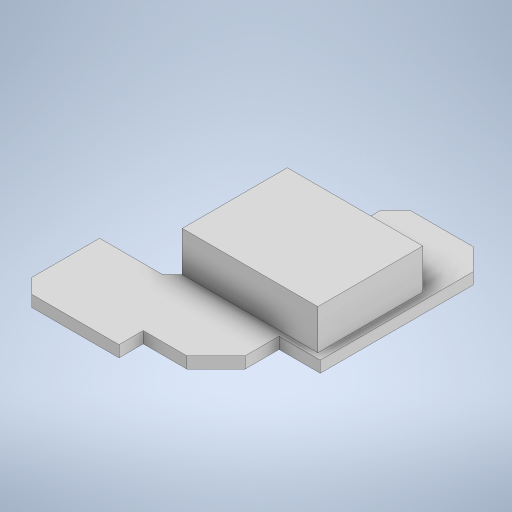
# Autodesk Inventor part: touch_pcb
Saved by Autodesk Inventor 2023 (Build 270158000, 158)
## iProperties
Created: 2023-03-12
Part Number: touch_pcb
Material: Generic
Document SubType Name: Modeling
Designer: nigel
Density: 1 g/cm^3
Appearance: Default
Author: nigel
Autodesk Inventor part; units mm, degrees
(part 1 of 2)
ref_plane "YZ Plane" through (0, 0, 0) normal (1, 0, 0) x (0, 1, 0)
ref_plane "XZ Plane" through (0, 0, 0) normal (0, 1, 0) x (-1, 0, 0)
sketch "Sketch1" plane through (0, 0, 0) normal (0, 1, 0) x (-1, 0, 0)
  arc A0 (8.4542, 10.3296) -> (8.3798, 10.2604) centre (8.417, 10.295) ccw
  arc A1 (10.1943, 12.5176) -> (10.1224, 12.5895) centre (10.1584, 12.5535) ccw
  arc A2 (8.7439, 11.2109) -> (8.8157, 11.1391) centre (8.7798, 11.175) ccw
  line L0 (10.1584, 12.5536) -> (8.7798, 11.175)
  arc A3 (8.7798, 11.1242) -> (8.7798, 11.2258) centre (8.7798, 11.175) ccw
  arc A4 (4.4414, 11.2258) -> (4.4414, 11.1242) centre (4.4414, 11.175) ccw
  line L1 (8.7798, 11.175) -> (4.4414, 11.175)
  arc A5 (4.4773, 11.1391) -> (4.4055, 11.2109) centre (4.4414, 11.175) ccw
  arc A6 (3.7865, 10.5919) -> (3.8583, 10.5201) centre (3.8224, 10.556) ccw
  line L2 (4.4414, 11.175) -> (3.8224, 10.556)
  arc A7 (3.8732, 10.556) -> (3.7716, 10.556) centre (3.8224, 10.556) ccw
  line L3 (3.8224, 10.556) -> (3.8224, 9.6448)
  arc A8 (10.1731, 10.4919) -> (10.1469, 10.5901) centre (10.16, 10.541) ccw
  arc A9 (9.053, 10.2987) -> (9.0792, 10.2005) centre (9.0661, 10.2496) ccw
  line L4 (10.16, 10.541) -> (9.0661, 10.2496)
  arc A10 (8.422, 10.215) -> (8.4964, 10.2842) centre (8.4592, 10.2496) ccw
  arc A11 (2.8503, 9.2057) -> (2.7785, 9.2775) centre (2.8144, 9.2416) ccw
  line L5 (8.4592, 10.2496) -> (8.417, 10.295)
  arc A12 (9.0661, 10.1988) -> (9.0661, 10.3004) centre (9.0661, 10.2496) ccw
  arc A13 (8.4592, 10.3004) -> (8.4592, 10.1988) centre (8.4592, 10.2496) ccw
  line L6 (9.0661, 10.2496) -> (8.4592, 10.2496)
  arc A14 (7.6178, 12.895) -> (7.5162, 12.895) centre (7.567, 12.895) ccw
  line L7 (7.567, 11.684) -> (7.567, 12.895)
  arc A15 (4.318, 11.7348) -> (4.318, 11.6332) centre (4.318, 11.684) ccw
  arc A16 (7.567, 11.6332) -> (7.567, 11.7348) centre (7.567, 11.684) ccw
  line L8 (4.318, 11.684) -> (7.567, 11.684)
  arc A17 (3.2781, 10.7159) -> (3.3499, 10.6441) centre (3.314, 10.68) ccw
  arc A18 (4.3539, 11.6481) -> (4.2821, 11.7199) centre (4.318, 11.684) ccw
  line L9 (3.314, 10.68) -> (4.318, 11.684)
  arc A19 (3.2632, 9.485) -> (3.3648, 9.485) centre (3.314, 9.485) ccw
  arc A20 (3.3648, 10.68) -> (3.2632, 10.68) centre (3.314, 10.68) ccw
  line L10 (3.314, 9.485) -> (3.314, 10.68)
  arc A21 (3.7716, 9.6448) -> (3.8732, 9.6448) centre (3.8224, 9.6448) ccw
  arc A22 (1.9961, 8.4951) -> (2.0679, 8.4233) centre (2.032, 8.4592) ccw
  line L11 (2.8144, 9.2416) -> (2.032, 8.4592)
  arc A23 (1.454, 1.1071) -> (1.5259, 1.1789) centre (1.4899, 1.143) ccw
  arc A24 (0.5852, 2.1196) -> (0.5134, 2.0477) centre (0.5493, 2.0837) ccw
  line L12 (1.49, 1.143) -> (0.5493, 2.0837)
  arc A25 (1.651, 1.0922) -> (1.651, 1.1938) centre (1.651, 1.143) ccw
  arc A26 (1.49, 1.1938) -> (1.49, 1.0922) centre (1.49, 1.143) ccw
  line L13 (1.651, 1.143) -> (1.49, 1.143)
  arc A27 (2.0679, 5.3321) -> (1.9961, 5.404) centre (2.032, 5.3681) ccw
  arc A28 (0.5134, 3.9213) -> (0.5852, 3.8494) centre (0.5493, 3.8854) ccw
  line L14 (2.032, 5.368) -> (0.5493, 3.8853)
  arc A29 (0.6001, 3.8853) -> (0.4985, 3.8853) centre (0.5493, 3.8853) ccw
  arc A30 (0.4985, 2.0837) -> (0.6001, 2.0837) centre (0.5493, 2.0837) ccw
  line L15 (0.5493, 3.8853) -> (0.5493, 2.0837)
  arc A31 (2.0828, 8.4592) -> (1.9812, 8.4592) centre (2.032, 8.4592) ccw
  arc A32 (1.9812, 5.368) -> (2.0828, 5.368) centre (2.032, 5.368) ccw
  line L16 (2.032, 8.4592) -> (2.032, 5.368)
  arc A33 (2.7636, 9.4427) -> (2.8652, 9.4437) centre (2.8144, 9.4432) ccw
  arc A34 (2.8648, 9.4855) -> (2.7632, 9.4845) centre (2.814, 9.485) ccw
  line L17 (2.8144, 9.4432) -> (2.814, 9.485)
  arc A35 (2.8652, 9.4432) -> (2.7636, 9.4432) centre (2.8144, 9.4432) ccw
  arc A36 (2.7636, 9.2416) -> (2.8652, 9.2416) centre (2.8144, 9.2416) ccw
  line L18 (2.8144, 9.4432) -> (2.8144, 9.2416)
  arc A37 (6.7529, 12.3511) -> (6.6811, 12.4229) centre (6.717, 12.387) ccw
  arc A38 (6.4025, 12.1443) -> (6.4743, 12.0725) centre (6.4384, 12.1084) ccw
  line L19 (6.717, 12.387) -> (6.4384, 12.1084)
  arc A39 (6.6662, 12.387) -> (6.7678, 12.387) centre (6.717, 12.387) ccw
  arc A40 (6.7678, 12.895) -> (6.6662, 12.895) centre (6.717, 12.895) ccw
  line L20 (6.717, 12.387) -> (6.717, 12.895)
  arc A41 (2.865, 10.9359) -> (2.7634, 10.9359) centre (2.8142, 10.9359) ccw
  arc A42 (2.7632, 9.485) -> (2.8648, 9.485) centre (2.814, 9.485) ccw
  line L21 (2.8142, 10.9359) -> (2.814, 9.485)
  arc A43 (4.019, 12.0725) -> (3.947, 12.1443) centre (3.983, 12.1084) ccw
  arc A44 (2.7782, 10.9717) -> (2.8502, 10.9) centre (2.8142, 10.9359) ccw
  line L22 (3.983, 12.1084) -> (2.8142, 10.9359)
  arc A45 (1.6151, 3.2109) -> (1.6869, 3.1391) centre (1.651, 3.175) ccw
  arc A46 (3.983, 12.1592) -> (3.983, 12.0576) centre (3.983, 12.1084) ccw
  line L23 (6.4384, 12.1084) -> (3.983, 12.1084)
  arc A47 (7.5162, 11.684) -> (7.6178, 11.684) centre (7.567, 11.684) ccw
  arc A48 (6.4384, 12.0576) -> (6.4384, 12.1592) centre (6.4384, 12.1084) ccw
  arc A49 (2.7696, 4.2218) -> (2.6978, 4.2936) centre (2.7337, 4.2577) ccw
  line L24 (2.7337, 4.2577) -> (1.651, 3.175)
  arc A50 (2.7845, 7.1723) -> (2.6829, 7.1723) centre (2.7337, 7.1723) ccw
  arc A51 (2.6829, 4.2577) -> (2.7845, 4.2577) centre (2.7337, 4.2577) ccw
  line L25 (2.7337, 7.1723) -> (2.7337, 4.2577)
  arc A52 (4.3499, 8.7167) -> (4.2781, 8.7885) centre (4.314, 8.7526) ccw
  arc A53 (2.6978, 7.2082) -> (2.7696, 7.1364) centre (2.7337, 7.1723) ccw
  line L26 (4.314, 8.7526) -> (2.7337, 7.1723)
  arc A54 (4.3648, 9.485) -> (4.2632, 9.485) centre (4.314, 9.485) ccw
  arc A55 (4.2632, 8.7526) -> (4.3648, 8.7526) centre (4.314, 8.7526) ccw
  line L27 (4.314, 9.485) -> (4.314, 8.7526)
  arc A56 (4.314, 10.3458) -> (4.314, 10.2442) centre (4.314, 10.295) ccw
  arc A57 (6.717, 10.2442) -> (6.717, 10.3458) centre (6.717, 10.295) ccw
  line L28 (4.314, 10.295) -> (6.717, 10.295)
  arc A58 (4.2632, 9.485) -> (4.3648, 9.485) centre (4.314, 9.485) ccw
  arc A59 (4.3648, 10.295) -> (4.2632, 10.295) centre (4.314, 10.295) ccw
  line L29 (4.314, 9.485) -> (4.314, 10.295)
  arc A60 (4.9689, 2.3571) -> (4.8971, 2.4289) centre (4.933, 2.393) ccw
  arc A61 (3.6471, 1.1789) -> (3.7189, 1.1071) centre (3.683, 1.143) ccw
  line L30 (4.933, 2.393) -> (3.683, 1.143)
  arc A62 (4.9838, 7.072) -> (4.8822, 7.072) centre (4.933, 7.072) ccw
  arc A63 (4.8822, 2.393) -> (4.9838, 2.393) centre (4.933, 2.393) ccw
  line L31 (4.933, 7.072) -> (4.933, 2.393)
  arc A64 (5.3499, 7.4171) -> (5.2781, 7.4889) centre (5.314, 7.453) ccw
  arc A65 (4.8971, 7.1079) -> (4.9689, 7.0361) centre (4.933, 7.072) ccw
  line L32 (5.314, 7.453) -> (4.933, 7.072)
  arc A66 (5.3648, 9.485) -> (5.2632, 9.485) centre (5.314, 9.485) ccw
  arc A67 (5.2632, 7.453) -> (5.3648, 7.453) centre (5.314, 7.453) ccw
  line L33 (5.314, 9.485) -> (5.314, 7.453)
  arc A68 (3.7338, 6.731) -> (3.6322, 6.731) centre (3.683, 6.731) ccw
  arc A69 (3.6322, 3.175) -> (3.7338, 3.175) centre (3.683, 3.175) ccw
  line L34 (3.683, 6.731) -> (3.683, 3.175)
  arc A70 (4.8663, 7.8425) -> (4.7945, 7.9143) centre (4.8304, 7.8784) ccw
  arc A71 (3.6471, 6.7669) -> (3.7189, 6.6951) centre (3.683, 6.731) ccw
  line L35 (4.8304, 7.8784) -> (3.683, 6.731)
  arc A72 (4.8812, 9.4686) -> (4.7796, 9.4686) centre (4.8304, 9.4686) ccw
  arc A73 (4.7796, 7.8784) -> (4.8812, 7.8784) centre (4.8304, 7.8784) ccw
  line L36 (4.8304, 9.4686) -> (4.8304, 7.8784)
  arc A74 (4.8499, 9.5209) -> (4.7781, 9.4491) centre (4.814, 9.485) ccw
  arc A75 (4.7945, 9.4327) -> (4.8663, 9.5045) centre (4.8304, 9.4686) ccw
  line L37 (4.814, 9.485) -> (4.8304, 9.4686)
  arc A76 (10.1077, 12.5578) -> (10.209, 12.5493) centre (10.1583, 12.5536) ccw
  arc A77 (10.2106, 12.5687) -> (10.1094, 12.5773) centre (10.16, 12.573) ccw
  line L38 (10.1584, 12.5536) -> (10.16, 12.573)
  arc A78 (3.8731, 9.6421) -> (3.7717, 9.6475) centre (3.8224, 9.6448) ccw
  arc A79 (3.7633, 9.4877) -> (3.8647, 9.4823) centre (3.814, 9.485) ccw
  line L39 (3.8224, 9.6448) -> (3.814, 9.485)
  line L40 (10.6689, 13.716) -> (11.43, 12.9549)
  line L41 (1.27, 0) -> (0.127, 1.143)
  line L42 (0.127, 1.143) -> (0.127, 9.144)
  line L43 (0.127, 9.144) -> (2.286, 9.144)
  line L44 (2.286, 9.144) -> (2.286, 10.922)
  line L45 (2.286, 10.922) -> (3.81, 12.446)
  line L46 (3.81, 12.446) -> (6.096, 12.446)
  line L47 (6.096, 12.446) -> (6.096, 13.716)
  line L48 (6.096, 13.716) -> (10.668, 13.716)
  arc A80 (2.159, 1.9431) -> (2.159, 1.8669) centre (2.159, 1.905) ccw
  arc A81 (2.413, 1.8669) -> (2.413, 1.9431) centre (2.413, 1.905) ccw
  line L49 (2.413, 0.635) -> (2.413, 0.381)
  arc A82 (2.3749, 0.381) -> (2.4511, 0.381) centre (2.413, 0.381) ccw
  arc A83 (2.4511, 0.635) -> (2.3749, 0.635) centre (2.413, 0.635) ccw
  line L50 (2.413, 0.381) -> (2.159, 0.381)
  arc A84 (2.159, 0.4191) -> (2.159, 0.3429) centre (2.159, 0.381) ccw
  arc A85 (2.413, 0.3429) -> (2.413, 0.4191) centre (2.413, 0.381) ccw
  line L51 (1.143, 0.381) -> (0.889, 0.381)
  arc A86 (0.889, 0.4191) -> (0.889, 0.3429) centre (0.889, 0.381) ccw
  arc A87 (1.143, 0.3429) -> (1.143, 0.4191) centre (1.143, 0.381) ccw
  line L52 (0.889, 0.381) -> (0.889, 0.635)
  arc A88 (0.9271, 0.635) -> (0.8509, 0.635) centre (0.889, 0.635) ccw
  arc A89 (0.8509, 0.381) -> (0.9271, 0.381) centre (0.889, 0.381) ccw
  line L53 (9.398, 11.811) -> (9.398, 12.065)
  arc A90 (9.652, 11.7729) -> (9.652, 11.8491) centre (9.652, 11.811) ccw
  arc A91 (9.398, 11.8491) -> (9.398, 11.7729) centre (9.398, 11.811) ccw
  line L54 (9.652, 11.811) -> (9.398, 11.811)
  arc A92 (0.514, 5.6358) -> (0.514, 5.5342) centre (0.514, 5.585) ccw
  arc A93 (7.614, 5.5342) -> (7.614, 5.6358) centre (7.614, 5.585) ccw
  line L55 (1.064, 5.485) -> (1.064, 4.085)
  arc A94 (1.0132, 4.085) -> (1.1148, 4.085) centre (1.064, 4.085) ccw
  arc A95 (1.1148, 5.485) -> (1.0132, 5.485) centre (1.064, 5.485) ccw
  line L56 (7.064, 5.485) -> (7.064, 4.085)
  arc A96 (7.0132, 4.085) -> (7.1148, 4.085) centre (7.064, 4.085) ccw
  arc A97 (7.1148, 5.485) -> (7.0132, 5.485) centre (7.064, 5.485) ccw
  line L57 (2.514, 3.885) -> (2.514, 3.485)
  arc A98 (2.4886, 3.485) -> (2.5394, 3.485) centre (2.514, 3.485) ccw
  arc A99 (2.5394, 3.885) -> (2.4886, 3.885) centre (2.514, 3.885) ccw
  line L58 (2.514, 3.485) -> (2.764, 3.735)
  arc A100 (2.782, 3.717) -> (2.746, 3.753) centre (2.764, 3.735) ccw
  arc A101 (2.496, 3.503) -> (2.532, 3.467) centre (2.514, 3.485) ccw
  line L59 (2.764, 3.735) -> (2.764, 3.885)
  arc A102 (2.7894, 3.885) -> (2.7386, 3.885) centre (2.764, 3.885) ccw
  arc A103 (2.7386, 3.735) -> (2.7894, 3.735) centre (2.764, 3.735) ccw
  arc A104 (1.9648, 7.985) -> (1.8632, 7.985) centre (1.914, 7.985) ccw
  arc A105 (1.8632, 5.735) -> (1.9648, 5.735) centre (1.914, 5.735) ccw
  arc A106 (2.064, 7.985) -> (1.914, 7.985) centre (1.989, 7.985) ccw
  arc A107 (2.0132, 7.985) -> (2.1148, 7.985) centre (2.064, 7.985) ccw
  arc A108 (1.8632, 7.985) -> (1.9648, 7.985) centre (1.914, 7.985) ccw
  line L60 (2.064, 7.985) -> (2.064, 5.735)
  arc A109 (2.0132, 5.735) -> (2.1148, 5.735) centre (2.064, 5.735) ccw
  arc A110 (2.1148, 7.985) -> (2.0132, 7.985) centre (2.064, 7.985) ccw
  line L61 (6.064, 5.735) -> (6.064, 7.985)
  arc A111 (6.1148, 7.985) -> (6.0132, 7.985) centre (6.064, 7.985) ccw
  arc A112 (6.0132, 5.735) -> (6.1148, 5.735) centre (6.064, 5.735) ccw
  arc A113 (6.214, 7.985) -> (6.064, 7.985) centre (6.139, 7.985) ccw
  arc A114 (6.1632, 7.985) -> (6.2648, 7.985) centre (6.214, 7.985) ccw
  arc A115 (6.0132, 7.985) -> (6.1148, 7.985) centre (6.064, 7.985) ccw
  line L62 (6.214, 7.985) -> (6.214, 5.735)
  arc A116 (6.1632, 5.735) -> (6.2648, 5.735) centre (6.214, 5.735) ccw
  arc A117 (6.2648, 7.985) -> (6.1632, 7.985) centre (6.214, 7.985) ccw
  line L63 (1.914, 5.735) -> (1.914, 7.985)
  arc A118 (10.922, 11.7729) -> (10.922, 11.8491) centre (10.922, 11.811) ccw
  arc A119 (10.668, 11.8491) -> (10.668, 11.7729) centre (10.668, 11.811) ccw
  line L64 (10.922, 11.811) -> (10.668, 11.811)
  arc A120 (10.9601, 12.065) -> (10.8839, 12.065) centre (10.922, 12.065) ccw
  arc A121 (10.8839, 11.811) -> (10.9601, 11.811) centre (10.922, 11.811) ccw
  line L65 (10.922, 12.065) -> (10.922, 11.811)
  arc A122 (10.922, 13.2969) -> (10.922, 13.3731) centre (10.922, 13.335) ccw
  arc A123 (10.668, 13.3731) -> (10.668, 13.2969) centre (10.668, 13.335) ccw
  line L66 (10.922, 13.335) -> (10.668, 13.335)
  arc A124 (10.9601, 13.335) -> (10.8839, 13.335) centre (10.922, 13.335) ccw
  arc A125 (10.8839, 13.081) -> (10.9601, 13.081) centre (10.922, 13.081) ccw
  line L67 (10.922, 13.335) -> (10.922, 13.081)
  arc A126 (9.3599, 9.779) -> (9.4361, 9.779) centre (9.398, 9.779) ccw
  arc A127 (9.4361, 10.033) -> (9.3599, 10.033) centre (9.398, 10.033) ccw
  line L68 (9.398, 9.779) -> (9.398, 10.033)
  arc A128 (9.652, 9.7409) -> (9.652, 9.8171) centre (9.652, 9.779) ccw
  line L69 (3.175, 2.413) -> (2.921, 2.413)
  arc A129 (9.398, 9.8171) -> (9.398, 9.7409) centre (9.398, 9.779) ccw
  line L70 (9.652, 9.779) -> (9.398, 9.779)
  arc A130 (10.922, 9.7409) -> (10.922, 9.8171) centre (10.922, 9.779) ccw
  arc A131 (10.668, 9.8171) -> (10.668, 9.7409) centre (10.668, 9.779) ccw
  line L71 (10.922, 9.779) -> (10.668, 9.779)
  arc A132 (10.9601, 10.033) -> (10.8839, 10.033) centre (10.922, 10.033) ccw
  arc A133 (10.8839, 9.779) -> (10.9601, 9.779) centre (10.922, 9.779) ccw
  line L72 (10.922, 10.033) -> (10.922, 9.779)
  arc A134 (10.922, 11.2649) -> (10.922, 11.3411) centre (10.922, 11.303) ccw
  arc A135 (10.668, 11.3411) -> (10.668, 11.2649) centre (10.668, 11.303) ccw
  line L73 (10.922, 11.303) -> (10.668, 11.303)
  arc A136 (10.9601, 11.303) -> (10.8839, 11.303) centre (10.922, 11.303) ccw
  arc A137 (10.8839, 11.049) -> (10.9601, 11.049) centre (10.922, 11.049) ccw
  line L74 (10.922, 11.303) -> (10.922, 11.049)
  arc A138 (9.4361, 11.303) -> (9.3599, 11.303) centre (9.398, 11.303) ccw
  arc A139 (9.3599, 11.049) -> (9.4361, 11.049) centre (9.398, 11.049) ccw
  line L75 (9.398, 11.303) -> (9.398, 11.049)
  arc A140 (9.398, 11.3411) -> (9.398, 11.2649) centre (9.398, 11.303) ccw
  arc A141 (9.652, 11.2649) -> (9.652, 11.3411) centre (9.652, 11.303) ccw
  line L76 (9.398, 11.303) -> (9.652, 11.303)
  line L77 (0.889, 1.905) -> (1.143, 1.905)
  arc A142 (1.143, 1.8669) -> (1.143, 1.9431) centre (1.143, 1.905) ccw
  arc A143 (0.889, 1.9431) -> (0.889, 1.8669) centre (0.889, 1.905) ccw
  line L78 (0.889, 1.905) -> (0.889, 1.651)
  arc A144 (0.8509, 1.651) -> (0.9271, 1.651) centre (0.889, 1.651) ccw
  arc A145 (0.9271, 1.905) -> (0.8509, 1.905) centre (0.889, 1.905) ccw
  line L79 (2.413, 1.905) -> (2.413, 1.651)
  arc A146 (2.3749, 1.651) -> (2.4511, 1.651) centre (2.413, 1.651) ccw
  arc A147 (2.4511, 1.905) -> (2.3749, 1.905) centre (2.413, 1.905) ccw
  line L80 (2.413, 1.905) -> (2.159, 1.905)
  arc A148 (9.4361, 12.065) -> (9.3599, 12.065) centre (9.398, 12.065) ccw
  arc A149 (9.3599, 11.811) -> (9.4361, 11.811) centre (9.398, 11.811) ccw
  line L81 (2.921, 3.937) -> (3.175, 3.937)
  arc A150 (3.175, 3.8989) -> (3.175, 3.9751) centre (3.175, 3.937) ccw
  arc A151 (2.921, 3.9751) -> (2.921, 3.8989) centre (2.921, 3.937) ccw
  line L82 (2.921, 3.937) -> (2.921, 3.683)
  arc A152 (2.8829, 3.683) -> (2.9591, 3.683) centre (2.921, 3.683) ccw
  arc A153 (2.9591, 3.937) -> (2.8829, 3.937) centre (2.921, 3.937) ccw
  line L83 (4.445, 3.937) -> (4.445, 3.683)
  arc A154 (4.4069, 3.683) -> (4.4831, 3.683) centre (4.445, 3.683) ccw
  arc A155 (4.4831, 3.937) -> (4.4069, 3.937) centre (4.445, 3.937) ccw
  line L84 (4.445, 3.937) -> (4.191, 3.937)
  arc A156 (4.191, 3.9751) -> (4.191, 3.8989) centre (4.191, 3.937) ccw
  arc A157 (4.445, 3.8989) -> (4.445, 3.9751) centre (4.445, 3.937) ccw
  line L85 (4.445, 2.667) -> (4.445, 2.413)
  arc A158 (4.4069, 2.413) -> (4.4831, 2.413) centre (4.445, 2.413) ccw
  arc A159 (4.4831, 2.667) -> (4.4069, 2.667) centre (4.445, 2.667) ccw
  line L86 (4.445, 2.413) -> (4.191, 2.413)
  arc A160 (4.191, 2.4511) -> (4.191, 2.3749) centre (4.191, 2.413) ccw
  arc A161 (4.445, 2.3749) -> (4.445, 2.4511) centre (4.445, 2.413) ccw
  arc A162 (2.921, 2.4511) -> (2.921, 2.3749) centre (2.921, 2.413) ccw
  arc A163 (3.175, 2.3749) -> (3.175, 2.4511) centre (3.175, 2.413) ccw
  line L87 (2.921, 2.413) -> (2.921, 2.667)
  arc A164 (2.9591, 2.667) -> (2.8829, 2.667) centre (2.921, 2.667) ccw
  arc A165 (2.8829, 2.413) -> (2.9591, 2.413) centre (2.921, 2.413) ccw
  line L88 (2.921, 1.905) -> (3.175, 1.905)
  arc A166 (3.175, 1.8669) -> (3.175, 1.9431) centre (3.175, 1.905) ccw
  arc A167 (2.921, 1.9431) -> (2.921, 1.8669) centre (2.921, 1.905) ccw
  line L89 (2.921, 1.905) -> (2.921, 1.651)
  arc A168 (2.8829, 1.651) -> (2.9591, 1.651) centre (2.921, 1.651) ccw
  arc A169 (2.9591, 1.905) -> (2.8829, 1.905) centre (2.921, 1.905) ccw
  line L90 (4.445, 1.905) -> (4.445, 1.651)
  arc A170 (4.4069, 1.651) -> (4.4831, 1.651) centre (4.445, 1.651) ccw
  arc A171 (4.4831, 1.905) -> (4.4069, 1.905) centre (4.445, 1.905) ccw
  line L91 (4.445, 1.905) -> (4.191, 1.905)
  arc A172 (4.191, 1.9431) -> (4.191, 1.8669) centre (4.191, 1.905) ccw
  arc A173 (4.445, 1.8669) -> (4.445, 1.9431) centre (4.445, 1.905) ccw
  line L92 (4.445, 0.635) -> (4.445, 0.381)
  arc A174 (4.4069, 0.381) -> (4.4831, 0.381) centre (4.445, 0.381) ccw
  arc A175 (4.4831, 0.635) -> (4.4069, 0.635) centre (4.445, 0.635) ccw
  line L93 (4.445, 0.381) -> (4.191, 0.381)
  arc A176 (4.191, 0.4191) -> (4.191, 0.3429) centre (4.191, 0.381) ccw
  arc A177 (4.445, 0.3429) -> (4.445, 0.4191) centre (4.445, 0.381) ccw
  line L94 (3.175, 0.381) -> (2.921, 0.381)
  arc A178 (2.921, 0.4191) -> (2.921, 0.3429) centre (2.921, 0.381) ccw
  arc A179 (3.175, 0.3429) -> (3.175, 0.4191) centre (3.175, 0.381) ccw
  line L95 (2.921, 0.381) -> (2.921, 0.635)
  arc A180 (2.9591, 0.635) -> (2.8829, 0.635) centre (2.921, 0.635) ccw
  arc A181 (2.8829, 0.381) -> (2.9591, 0.381) centre (2.921, 0.381) ccw
  line L96 (9.017, 10.795) -> (6.117, 10.795)
  arc A182 (6.117, 10.8268) -> (6.117, 10.7632) centre (6.117, 10.795) ccw
  arc A183 (9.017, 10.7632) -> (9.017, 10.8268) centre (9.017, 10.795) ccw
  line L97 (9.017, 10.795) -> (9.017, 12.395)
  arc A184 (8.9853, 10.795) -> (9.0488, 10.795) centre (9.0171, 10.795) ccw
  line L98 (9.017, 12.395) -> (6.117, 12.395)
  arc A185 (6.117, 12.4268) -> (6.117, 12.3633) centre (6.117, 12.3951) ccw
  arc A186 (9.017, 12.3633) -> (9.017, 12.4268) centre (9.017, 12.3951) ccw
  line L99 (6.117, 12.395) -> (6.117, 10.795)
  arc A187 (6.0853, 10.795) -> (6.1487, 10.795) centre (6.117, 10.795) ccw
  arc A188 (6.1487, 12.395) -> (6.0853, 12.395) centre (6.117, 12.395) ccw
  line L100 (0.889, 3.937) -> (1.143, 3.937)
  arc A189 (1.143, 3.8989) -> (1.143, 3.9751) centre (1.143, 3.937) ccw
  arc A190 (0.889, 3.9751) -> (0.889, 3.8989) centre (0.889, 3.937) ccw
  line L101 (0.889, 3.937) -> (0.889, 3.683)
  arc A191 (0.8509, 3.683) -> (0.9271, 3.683) centre (0.889, 3.683) ccw
  arc A192 (0.9271, 3.937) -> (0.8509, 3.937) centre (0.889, 3.937) ccw
  line L102 (2.413, 3.937) -> (2.413, 3.683)
  arc A193 (2.3749, 3.683) -> (2.4511, 3.683) centre (2.413, 3.683) ccw
  arc A194 (2.4511, 3.937) -> (2.3749, 3.937) centre (2.413, 3.937) ccw
  line L103 (2.413, 3.937) -> (2.159, 3.937)
  arc A195 (2.159, 3.9751) -> (2.159, 3.8989) centre (2.159, 3.937) ccw
  arc A196 (2.413, 3.8989) -> (2.413, 3.9751) centre (2.413, 3.937) ccw
  line L104 (2.413, 2.667) -> (2.413, 2.413)
  arc A197 (2.3749, 2.413) -> (2.4511, 2.413) centre (2.413, 2.413) ccw
  arc A198 (2.4511, 2.667) -> (2.3749, 2.667) centre (2.413, 2.667) ccw
  line L105 (2.413, 2.413) -> (2.159, 2.413)
  arc A199 (2.159, 2.4511) -> (2.159, 2.3749) centre (2.159, 2.413) ccw
  arc A200 (2.413, 2.3749) -> (2.413, 2.4511) centre (2.413, 2.413) ccw
  line L106 (1.143, 2.413) -> (0.889, 2.413)
  arc A201 (0.889, 2.4511) -> (0.889, 2.3749) centre (0.889, 2.413) ccw
  arc A202 (1.143, 2.3749) -> (1.143, 2.4511) centre (1.143, 2.413) ccw
  line L107 (0.889, 2.413) -> (0.889, 2.667)
  arc A203 (0.9271, 2.667) -> (0.8509, 2.667) centre (0.889, 2.667) ccw
  arc A204 (0.8509, 2.413) -> (0.9271, 2.413) centre (0.889, 2.413) ccw
  line L108 (2.314, 5.735) -> (2.314, 5.785)
  arc A205 (2.3394, 5.785) -> (2.2886, 5.785) centre (2.314, 5.785) ccw
  arc A206 (2.2886, 5.735) -> (2.3394, 5.735) centre (2.314, 5.735) ccw
  line L109 (2.314, 5.785) -> (2.564, 6.135)
  arc A207 (2.5847, 6.1202) -> (2.5433, 6.1498) centre (2.564, 6.135) ccw
  arc A208 (2.2933, 5.7998) -> (2.3347, 5.7702) centre (2.314, 5.785) ccw
  line L110 (2.564, 6.135) -> (2.814, 5.785)
  arc A209 (2.7933, 5.7702) -> (2.8347, 5.7998) centre (2.814, 5.785) ccw
  arc A210 (2.5847, 6.1498) -> (2.5433, 6.1202) centre (2.564, 6.135) ccw
  line L111 (2.814, 5.785) -> (2.814, 5.735)
  arc A211 (2.7886, 5.735) -> (2.8394, 5.735) centre (2.814, 5.735) ccw
  arc A212 (2.8394, 5.785) -> (2.7886, 5.785) centre (2.814, 5.785) ccw
  line L112 (2.814, 5.735) -> (2.314, 5.735)
  arc A213 (2.314, 5.7604) -> (2.314, 5.7096) centre (2.314, 5.735) ccw
  arc A214 (2.814, 5.7096) -> (2.814, 5.7604) centre (2.814, 5.735) ccw
  line L113 (2.3184, 5.7912) -> (2.8096, 5.7912)
  arc A215 (2.8096, 5.7658) -> (2.8096, 5.8166) centre (2.8096, 5.7912) ccw
  arc A216 (2.3184, 5.8166) -> (2.3184, 5.7658) centre (2.3184, 5.7912) ccw
  line L114 (2.391, 5.8928) -> (2.737, 5.8928)
  arc A217 (2.737, 5.8674) -> (2.737, 5.9182) centre (2.737, 5.8928) ccw
  arc A218 (2.391, 5.9182) -> (2.391, 5.8674) centre (2.391, 5.8928) ccw
  line L115 (2.4636, 5.9944) -> (2.6644, 5.9944)
  arc A219 (2.6644, 5.969) -> (2.6644, 6.0198) centre (2.6644, 5.9944) ccw
  arc A220 (2.4636, 6.0198) -> (2.4636, 5.969) centre (2.4636, 5.9944) ccw
  line L116 (2.5361, 6.096) -> (2.5919, 6.096)
  arc A221 (2.5919, 6.0706) -> (2.5919, 6.1214) centre (2.5919, 6.096) ccw
  arc A222 (2.5361, 6.1214) -> (2.5361, 6.0706) centre (2.5361, 6.096) ccw
  line L117 (-0.386, 3.985) -> (-0.386, 3.485)
  arc A223 (-0.4368, 3.485) -> (-0.3352, 3.485) centre (-0.386, 3.485) ccw
  arc A224 (-0.3352, 3.985) -> (-0.4368, 3.985) centre (-0.386, 3.985) ccw
  line L118 (-0.386, 3.485) -> (-0.286, 3.385)
  arc A225 (-0.3219, 3.3491) -> (-0.2501, 3.4209) centre (-0.286, 3.385) ccw
  arc A226 (-0.3501, 3.5209) -> (-0.4219, 3.4491) centre (-0.386, 3.485) ccw
  line L119 (-0.286, 3.385) -> (8.414, 3.385)
  arc A227 (-0.286, 3.4358) -> (-0.286, 3.3342) centre (-0.286, 3.385) ccw
  line L120 (8.414, 3.385) -> (8.514, 3.485)
  line L121 (8.514, 3.485) -> (8.514, 3.985)
  arc A228 (8.5648, 3.985) -> (8.4632, 3.985) centre (8.514, 3.985) ccw
  line L122 (8.514, 3.985) -> (-0.386, 3.985)
  arc A229 (-0.386, 4.0358) -> (-0.386, 3.9342) centre (-0.386, 3.985) ccw
  arc A230 (8.514, 3.9342) -> (8.514, 4.0358) centre (8.514, 3.985) ccw
  line L123 (7.614, 5.585) -> (0.514, 5.585)
  arc A231 (2.266, 4.8327) -> (2.2298, 4.8447) centre (2.2479, 4.8387) ccw
  line L124 (3.4452, 4.1021) -> (3.1178, 4.1021)
  arc A232 (3.4643, 4.8387) -> (3.4262, 4.8387) centre (3.4453, 4.8387) ccw
  arc A233 (3.4262, 4.1021) -> (3.4643, 4.1021) centre (3.4453, 4.1021) ccw
  line L125 (3.4452, 4.8387) -> (3.4452, 4.1021)
  arc A234 (3.9194, 4.8197) -> (3.9194, 4.8578) centre (3.9194, 4.8388) ccw
  arc A235 (3.7557, 4.8578) -> (3.7557, 4.8197) centre (3.7557, 4.8388) ccw
  line L126 (3.9194, 4.8387) -> (3.7557, 4.8387)
  arc A236 (3.9194, 4.8577) -> (3.9194, 4.8196) centre (3.9194, 4.8387) ccw
  arc A237 (4.064, 4.675) -> (4.1021, 4.675) centre (4.0831, 4.675) ccw
  arc A238 (4.0831, 4.675) -> (3.9194, 4.8387) centre (3.9194, 4.675) ccw
  arc A239 (4.064, 4.2658) -> (4.1021, 4.2658) centre (4.0831, 4.2658) ccw
  arc A240 (4.1021, 4.675) -> (4.064, 4.675) centre (4.0831, 4.675) ccw
  line L127 (4.0831, 4.2658) -> (4.0831, 4.675)
  arc A241 (4.1021, 4.2658) -> (4.064, 4.2658) centre (4.0831, 4.2658) ccw
  arc A242 (3.9194, 4.1212) -> (3.9194, 4.0831) centre (3.9194, 4.1021) ccw
  arc A243 (3.9194, 4.1021) -> (4.0831, 4.2658) centre (3.9194, 4.2658) ccw
  arc A244 (3.7557, 4.1212) -> (3.7557, 4.0831) centre (3.7557, 4.1021) ccw
  line L128 (2.2479, 4.8387) -> (2.0024, 4.1021)
  arc A245 (1.9843, 4.1081) -> (2.0204, 4.0961) centre (2.0023, 4.1021) ccw
  arc A246 (4.4082, 4.7926) -> (4.431, 4.7621) centre (4.4196, 4.7774) ccw
  line L129 (2.0024, 4.1021) -> (1.7568, 4.8387)
  arc A247 (1.7749, 4.8447) -> (1.7388, 4.8327) centre (1.7569, 4.8387) ccw
  arc A248 (1.9843, 4.0961) -> (2.0204, 4.1081) centre (2.0023, 4.1021) ccw
  line L130 (1.4676, 4.3886) -> (0.9766, 4.3886)
  arc A249 (0.9766, 4.4076) -> (0.9766, 4.3695) centre (0.9766, 4.3886) ccw
  arc A250 (1.4676, 4.3695) -> (1.4676, 4.4076) centre (1.4676, 4.3886) ccw
  line L131 (1.2221, 4.143) -> (1.2221, 4.6341)
  arc A251 (1.2411, 4.6341) -> (1.203, 4.6341) centre (1.2221, 4.6341) ccw
  arc A252 (1.203, 4.143) -> (1.2411, 4.143) centre (1.2221, 4.143) ccw
  arc A253 (4.3787, 4.2658) -> (4.5424, 4.1021) centre (4.5424, 4.2658) ccw
  arc A254 (4.3977, 4.2658) -> (4.3596, 4.2658) centre (4.3787, 4.2658) ccw
  arc A255 (4.5424, 4.0831) -> (4.5424, 4.1211) centre (4.5424, 4.1021) ccw
  arc A256 (4.5424, 4.1021) -> (4.7879, 4.2044) centre (4.5424, 4.4478) ccw
  arc A257 (4.5424, 4.1211) -> (4.5424, 4.0831) centre (4.5424, 4.1021) ccw
  arc A258 (4.8014, 4.191) -> (4.7744, 4.2178) centre (4.7879, 4.2044) ccw
  arc A259 (4.7674, 4.675) -> (4.6037, 4.8387) centre (4.6037, 4.675) ccw
  arc A260 (4.7484, 4.675) -> (4.7865, 4.675) centre (4.7675, 4.675) ccw
  arc A261 (4.6037, 4.8578) -> (4.6037, 4.8197) centre (4.6037, 4.8388) ccw
  arc A262 (4.6038, 4.8197) -> (4.6037, 4.8577) centre (4.6037, 4.8387) ccw
  arc A263 (3.9194, 4.0831) -> (3.9194, 4.1212) centre (3.9194, 4.1021) ccw
  arc A264 (4.6856, 4.5318) -> (4.7674, 4.675) centre (4.6012, 4.675) ccw
  arc A265 (4.6759, 4.5482) -> (4.6953, 4.5154) centre (4.6856, 4.5318) ccw
  arc A266 (4.7865, 4.675) -> (4.7484, 4.675) centre (4.7675, 4.675) ccw
  line L132 (3.7557, 4.1021) -> (3.9194, 4.1021)
  arc A267 (4.4514, 4.4257) -> (4.4696, 4.3923) centre (4.4605, 4.409) ccw
  arc A268 (4.6947, 4.5151) -> (4.6765, 4.5485) centre (4.6856, 4.5318) ccw
  line L133 (4.4605, 4.409) -> (4.6856, 4.5318)
  arc A269 (4.3596, 4.2658) -> (4.3977, 4.2658) centre (4.3787, 4.2658) ccw
  arc A270 (4.4702, 4.3926) -> (4.4509, 4.4254) centre (4.4605, 4.409) ccw
  arc A271 (4.4605, 4.409) -> (4.3787, 4.2658) centre (4.5449, 4.2658) ccw
  arc A272 (9.1059, 10.9157) -> (9.1059, 10.9538) centre (9.1059, 10.9347) ccw
  arc A273 (8.9422, 10.9538) -> (8.9422, 10.9157) centre (8.9422, 10.9347) ccw
  line L134 (9.1059, 10.9347) -> (8.9422, 10.9347)
  arc A274 (9.1059, 10.1791) -> (9.1059, 10.2172) centre (9.1059, 10.1982) ccw
  arc A275 (8.9422, 10.2172) -> (8.9422, 10.1791) centre (8.9422, 10.1982) ccw
  line L135 (9.1059, 10.1981) -> (8.9422, 10.1981)
  arc A276 (9.0431, 10.9347) -> (9.005, 10.9347) centre (9.0241, 10.9347) ccw
  arc A277 (9.005, 10.1981) -> (9.0431, 10.1981) centre (9.0241, 10.1981) ccw
  line L136 (9.0241, 10.9347) -> (9.0241, 10.1981)
  arc A278 (8.0674, 12.5537) -> (8.0856, 12.5203) centre (8.0765, 12.537) ccw
  arc A279 (7.9756, 12.3938) -> (8.0137, 12.3938) centre (7.9947, 12.3938) ccw
  arc A280 (8.0862, 12.5206) -> (8.0668, 12.5534) centre (8.0765, 12.537) ccw
  arc A281 (8.0765, 12.537) -> (7.9947, 12.3938) centre (8.1609, 12.3938) ccw
  arc A282 (4.6037, 4.8387) -> (4.4196, 4.7773) centre (4.6037, 4.5319) ccw
  arc A283 (8.0137, 12.3938) -> (7.9756, 12.3938) centre (7.9947, 12.3938) ccw
  arc A284 (8.8774, 12.549) -> (8.8433, 12.566) centre (8.8604, 12.5575) ccw
  arc A285 (8.9013, 12.5765) -> (8.9013, 12.5384) centre (8.9013, 12.5575) ccw
  arc A286 (9.1059, 12.5384) -> (9.1059, 12.5765) centre (9.1059, 12.5575) ccw
  arc A287 (8.9013, 12.5384) -> (8.9013, 12.5765) centre (8.9013, 12.5575) ccw
  arc A288 (8.9013, 12.9477) -> (8.9013, 12.9858) centre (8.9013, 12.9668) ccw
  arc A289 (8.9013, 12.9858) -> (8.9013, 12.9477) centre (8.9013, 12.9668) ccw
  arc A290 (9.0869, 12.2301) -> (9.125, 12.2301) centre (9.1059, 12.2301) ccw
  arc A291 (0.8142, 2.5337) -> (0.8142, 2.5718) centre (0.8142, 2.5528) ccw
  arc A292 (0.5687, 2.5718) -> (0.5687, 2.5337) centre (0.5687, 2.5528) ccw
  line L137 (0.8142, 2.5527) -> (0.5687, 2.5527)
  arc A293 (0.8142, 2.5717) -> (0.8142, 2.5336) centre (0.8142, 2.5527) ccw
  arc A294 (0.9588, 2.389) -> (0.997, 2.389) centre (0.9779, 2.389) ccw
  arc A295 (0.9779, 2.389) -> (0.8142, 2.5527) centre (0.8142, 2.389) ccw
  arc A296 (0.9588, 1.9798) -> (0.997, 1.9798) centre (0.9779, 1.9798) ccw
  arc A297 (0.997, 2.389) -> (0.9588, 2.389) centre (0.9779, 2.389) ccw
  line L138 (0.9779, 1.9798) -> (0.9779, 2.389)
  arc A298 (0.997, 1.9798) -> (0.9588, 1.9798) centre (0.9779, 1.9798) ccw
  arc A299 (0.8142, 1.8352) -> (0.8142, 1.7971) centre (0.8142, 1.8161) ccw
  arc A300 (0.8142, 1.8161) -> (0.9779, 1.9798) centre (0.8142, 1.9798) ccw
  arc A301 (0.5687, 1.8352) -> (0.5687, 1.7971) centre (0.5687, 1.8161) ccw
  arc A302 (0.8142, 1.7971) -> (0.8142, 1.8352) centre (0.8142, 1.8161) ccw
  line L139 (0.5687, 1.8161) -> (0.8142, 1.8161)
  arc A303 (0.5877, 2.2253) -> (0.5496, 2.2253) centre (0.5686, 2.2253) ccw
  arc A304 (0.5496, 1.8161) -> (0.5877, 1.8161) centre (0.5686, 1.8161) ccw
  line L140 (0.5687, 2.2253) -> (0.5687, 1.8161)
  arc A305 (0.6914, 2.2063) -> (0.6914, 2.2444) centre (0.6914, 2.2254) ccw
  arc A306 (0.5687, 2.2444) -> (0.5687, 2.2063) centre (0.5687, 2.2254) ccw
  line L141 (0.6914, 2.2253) -> (0.5687, 2.2253)
  arc A307 (3.4452, 4.0831) -> (3.4452, 4.1212) centre (3.4452, 4.1021) ccw
  arc A308 (3.1178, 4.1212) -> (3.1178, 4.0831) centre (3.1178, 4.1021) ccw
  arc A309 (8.128, 9.4234) -> (8.128, 9.3726) centre (8.128, 9.398) ccw
  line L142 (8.128, 9.398) -> (7.62, 8.89)
  arc A310 (7.602, 8.908) -> (7.638, 8.872) centre (7.62, 8.89) ccw
  arc A311 (8.146, 9.38) -> (8.11, 9.416) centre (8.128, 9.398) ccw
  line L143 (7.62, 8.89) -> (7.62, 5.588)
  arc A312 (7.5946, 5.588) -> (7.6454, 5.588) centre (7.62, 5.588) ccw
  arc A313 (7.6454, 8.89) -> (7.5946, 8.89) centre (7.62, 8.89) ccw
  line L144 (7.62, 5.588) -> (5.334, 5.588)
  arc A314 (5.334, 5.6134) -> (5.334, 5.5626) centre (5.334, 5.588) ccw
  arc A315 (7.62, 5.5626) -> (7.62, 5.6134) centre (7.62, 5.588) ccw
  line L145 (5.334, 5.588) -> (5.334, 0.762)
  arc A316 (5.3086, 0.762) -> (5.3594, 0.762) centre (5.334, 0.762) ccw
  arc A317 (5.3594, 5.588) -> (5.3086, 5.588) centre (5.334, 5.588) ccw
  line L146 (5.334, 0.762) -> (4.572, 0)
  arc A318 (4.554, 0.018) -> (4.59, -0.018) centre (4.572, 0) ccw
  arc A319 (5.352, 0.744) -> (5.316, 0.78) centre (5.334, 0.762) ccw
  line L147 (11.43, 9.398) -> (8.128, 9.398)
  line L148 (1.5113, 7.4078) -> (2.2479, 7.6533)
  arc A320 (2.2539, 7.6352) -> (2.2419, 7.6714) centre (2.2479, 7.6533) ccw
  arc A321 (1.5053, 7.4258) -> (1.5173, 7.3897) centre (1.5113, 7.4078) ccw
  line L149 (2.0842, 7.9347) -> (2.2479, 8.1393)
  arc A322 (2.2628, 8.1274) -> (2.233, 8.1512) centre (2.2479, 8.1393) ccw
  arc A323 (2.0693, 7.9466) -> (2.0991, 7.9228) centre (2.0842, 7.9347) ccw
  line L150 (2.2479, 8.1393) -> (1.5113, 8.1393)
  arc A324 (1.5113, 8.1583) -> (1.5113, 8.1202) centre (1.5113, 8.1393) ccw
  arc A325 (2.2479, 8.1202) -> (2.2479, 8.1583) centre (2.2479, 8.1393) ccw
  line L151 (1.5113, 7.9347) -> (1.5113, 8.3439)
  arc A326 (1.5304, 8.3439) -> (1.4923, 8.3439) centre (1.5114, 8.3439) ccw
  arc A327 (1.4923, 7.9347) -> (1.5304, 7.9347) centre (1.5114, 7.9347) ccw
  line L152 (11.43, 9.398) -> (8.128, 9.398)
  arc A328 (8.128, 9.4234) -> (8.128, 9.3726) centre (8.128, 9.398) ccw
  line L153 (8.128, 9.398) -> (7.62, 8.89)
  arc A329 (7.602, 8.908) -> (7.638, 8.872) centre (7.62, 8.89) ccw
  arc A330 (8.146, 9.38) -> (8.11, 9.416) centre (8.128, 9.398) ccw
  line L154 (7.62, 8.89) -> (7.62, 5.588)
  arc A331 (7.5946, 5.588) -> (7.6454, 5.588) centre (7.62, 5.588) ccw
  arc A332 (7.6454, 8.89) -> (7.5946, 8.89) centre (7.62, 8.89) ccw
  line L155 (7.62, 5.588) -> (5.334, 5.588)
  arc A333 (5.334, 5.6134) -> (5.334, 5.5626) centre (5.334, 5.588) ccw
  arc A334 (7.62, 5.5626) -> (7.62, 5.6134) centre (7.62, 5.588) ccw
  line L156 (5.334, 5.588) -> (5.334, 0.762)
  arc A335 (5.3086, 0.762) -> (5.3594, 0.762) centre (5.334, 0.762) ccw
  arc A336 (5.3594, 5.588) -> (5.3086, 5.588) centre (5.334, 5.588) ccw
  line L157 (5.334, 0.762) -> (4.572, 0)
  arc A337 (4.554, 0.018) -> (4.59, -0.018) centre (4.572, 0) ccw
  arc A338 (5.352, 0.744) -> (5.316, 0.78) centre (5.334, 0.762) ccw
  line L158 (4.0513, 5.5767) -> (4.7879, 5.5767)
  arc A339 (4.7879, 5.5577) -> (4.7879, 5.5958) centre (4.7879, 5.5768) ccw
  arc A340 (4.0513, 5.5958) -> (4.0513, 5.5577) centre (4.0513, 5.5768) ccw
  line L159 (4.7879, 5.3721) -> (4.7879, 5.7813)
  arc A341 (4.807, 5.7813) -> (4.7689, 5.7813) centre (4.788, 5.7813) ccw
  arc A342 (4.7689, 5.3721) -> (4.807, 5.3721) centre (4.788, 5.3721) ccw
  line L160 (4.215, 6.047) -> (4.3787, 6.047)
  arc A343 (4.3787, 6.028) -> (4.3787, 6.0661) centre (4.3787, 6.0471) ccw
  arc A344 (4.215, 6.0661) -> (4.215, 6.028) centre (4.215, 6.0471) ccw
  arc A345 (4.3787, 6.047) -> (4.3787, 6.3744) centre (4.3787, 6.2107) ccw
  arc A346 (4.3787, 6.0661) -> (4.3787, 6.028) centre (4.3787, 6.0471) ccw
  arc A347 (4.3787, 6.3934) -> (4.3787, 6.3553) centre (4.3787, 6.3743) ccw
  line L161 (4.3787, 6.3744) -> (4.215, 6.3744)
  arc A348 (4.215, 6.3934) -> (4.215, 6.3553) centre (4.215, 6.3743) ccw
  arc A349 (4.3787, 6.3553) -> (4.3787, 6.3934) centre (4.3787, 6.3743) ccw
  arc A350 (4.215, 6.3744) -> (4.215, 6.047) centre (4.215, 6.2107) ccw
  arc A351 (4.215, 6.3553) -> (4.215, 6.3934) centre (4.215, 6.3743) ccw
  arc A352 (4.215, 6.028) -> (4.215, 6.0661) centre (4.215, 6.0471) ccw
  line L162 (4.5424, 6.7054) -> (4.1741, 6.7054)
  arc A353 (4.1741, 6.7244) -> (4.1741, 6.6863) centre (4.1741, 6.7054) ccw
  arc A354 (4.5424, 6.6863) -> (4.5424, 6.7244) centre (4.5424, 6.7054) ccw
  arc A355 (4.0513, 6.8281) -> (4.1741, 6.7054) centre (4.1741, 6.8282) ccw
  arc A356 (4.0704, 6.8281) -> (4.0323, 6.8281) centre (4.0514, 6.8281) ccw
  arc A357 (4.1741, 6.6863) -> (4.1741, 6.7244) centre (4.1741, 6.7054) ccw
  line L163 (4.0513, 6.8281) -> (4.0513, 7.0327)
  arc A358 (4.0704, 7.0327) -> (4.0323, 7.0327) centre (4.0514, 7.0327) ccw
  arc A359 (4.0323, 6.8281) -> (4.0704, 6.8281) centre (4.0514, 6.8281) ccw
  line L164 (4.0513, 7.0327) -> (4.5424, 7.0327)
  arc A360 (4.5424, 7.0137) -> (4.5424, 7.0518) centre (4.5424, 7.0328) ccw
  arc A361 (4.0513, 7.0518) -> (4.0513, 7.0137) centre (4.0513, 7.0328) ccw
  line L165 (4.0513, 7.6511) -> (4.0513, 7.4874)
  arc A362 (4.0323, 7.4874) -> (4.0704, 7.4874) centre (4.0514, 7.4874) ccw
  arc A363 (4.0704, 7.6511) -> (4.0323, 7.6511) centre (4.0514, 7.6511) ccw
  arc A364 (4.0513, 7.4874) -> (4.1741, 7.3647) centre (4.1741, 7.4875) ccw
  arc A365 (4.0704, 7.4874) -> (4.0323, 7.4874) centre (4.0514, 7.4874) ccw
  arc A366 (4.1741, 7.3456) -> (4.1741, 7.3837) centre (4.1741, 7.3647) ccw
  line L166 (4.1741, 7.3647) -> (4.4196, 7.3647)
  arc A367 (4.4196, 7.3456) -> (4.4196, 7.3837) centre (4.4196, 7.3647) ccw
  arc A368 (4.1741, 7.3837) -> (4.1741, 7.3456) centre (4.1741, 7.3647) ccw
  arc A369 (4.4196, 7.3647) -> (4.5424, 7.4874) centre (4.4196, 7.4875) ccw
  arc A370 (4.4196, 7.3837) -> (4.4196, 7.3456) centre (4.4196, 7.3647) ccw
  arc A371 (4.5614, 7.4874) -> (4.5233, 7.4874) centre (4.5423, 7.4874) ccw
  line L167 (4.5424, 7.4874) -> (4.5424, 7.6511)
  arc A372 (4.5614, 7.6511) -> (4.5233, 7.6511) centre (4.5423, 7.6511) ccw
  arc A373 (4.5233, 7.4874) -> (4.5614, 7.4874) centre (4.5423, 7.4874) ccw
  line L168 (4.0513, 7.9489) -> (4.7879, 7.9489)
  arc A374 (4.7879, 7.9299) -> (4.7879, 7.968) centre (4.7879, 7.9489) ccw
  arc A375 (4.0513, 7.968) -> (4.0513, 7.9299) centre (4.0513, 7.9489) ccw
  line L169 (4.5424, 7.9489) -> (4.5424, 8.1536)
  arc A376 (4.5614, 8.1536) -> (4.5233, 8.1536) centre (4.5423, 8.1536) ccw
  arc A377 (4.5233, 7.9489) -> (4.5614, 7.9489) centre (4.5423, 7.9489) ccw
  arc A378 (4.5424, 8.1536) -> (4.4196, 8.2763) centre (4.4196, 8.1535) ccw
  arc A379 (4.5233, 8.1536) -> (4.5614, 8.1536) centre (4.5423, 8.1536) ccw
  arc A380 (4.4196, 8.2954) -> (4.4196, 8.2573) centre (4.4196, 8.2764) ccw
  line L170 (4.4196, 8.2763) -> (4.0513, 8.2763)
  arc A381 (4.0513, 8.2954) -> (4.0513, 8.2573) centre (4.0513, 8.2764) ccw
  arc A382 (4.4196, 8.2573) -> (4.4196, 8.2954) centre (4.4196, 8.2764) ccw
  line L171 (4.2559, 8.8733) -> (4.3378, 8.6687)
  arc A383 (4.3201, 8.6616) -> (4.3554, 8.6758) centre (4.3377, 8.6687) ccw
  arc A384 (4.2736, 8.8804) -> (4.2382, 8.8662) centre (4.2559, 8.8733) ccw
  arc A385 (4.3378, 8.6687) -> (4.5424, 8.7096) centre (4.4363, 8.7081) ccw
  arc A386 (4.3554, 8.6758) -> (4.3201, 8.6616) centre (4.3377, 8.6687) ccw
  arc A387 (4.5614, 8.7099) -> (4.5233, 8.7093) centre (4.5423, 8.7096) ccw
  arc A388 (4.5424, 8.7096) -> (4.5014, 8.8938) centre (4.0774, 8.7028) ccw
  arc A389 (4.5233, 8.7093) -> (4.5614, 8.7099) centre (4.5423, 8.7096) ccw
  arc A390 (4.5188, 8.9016) -> (4.4841, 8.8859) centre (4.5015, 8.8938) ccw
  arc A391 (4.2559, 8.8733) -> (4.0513, 8.8324) centre (4.1574, 8.8339) ccw
  arc A392 (4.2382, 8.8662) -> (4.2736, 8.8804) centre (4.2559, 8.8733) ccw
  arc A393 (4.0322, 8.8321) -> (4.0703, 8.8327) centre (4.0512, 8.8324) ccw
  arc A394 (4.0513, 8.8324) -> (4.0922, 8.6073) centre (4.7451, 8.8422) ccw
  arc A395 (4.0703, 8.8327) -> (4.0323, 8.8321) centre (4.0513, 8.8324) ccw
  arc A396 (4.0743, 8.6009) -> (4.1101, 8.6138) centre (4.0922, 8.6074) ccw
  line L172 (4.0513, 9.5287) -> (4.0513, 9.365)
  arc A397 (4.0323, 9.365) -> (4.0704, 9.365) centre (4.0514, 9.365) ccw
  arc A398 (4.0704, 9.5287) -> (4.0323, 9.5287) centre (4.0514, 9.5287) ccw
  arc A399 (4.0513, 9.365) -> (4.1741, 9.2422) centre (4.1741, 9.365) ccw
  arc A400 (4.0704, 9.365) -> (4.0323, 9.365) centre (4.0514, 9.365) ccw
  arc A401 (4.1741, 9.2232) -> (4.1741, 9.2613) centre (4.1741, 9.2423) ccw
  line L173 (4.1741, 9.2422) -> (4.4196, 9.2422)
  arc A402 (4.4196, 9.2232) -> (4.4196, 9.2613) centre (4.4196, 9.2423) ccw
  arc A403 (4.1741, 9.2613) -> (4.1741, 9.2232) centre (4.1741, 9.2423) ccw
  arc A404 (4.4196, 9.2422) -> (4.5424, 9.365) centre (4.4196, 9.365) ccw
  arc A405 (4.4196, 9.2613) -> (4.4196, 9.2232) centre (4.4196, 9.2423) ccw
  arc A406 (4.5614, 9.365) -> (4.5233, 9.365) centre (4.5423, 9.365) ccw
  line L174 (4.5424, 9.365) -> (4.5424, 9.5287)
  arc A407 (4.5614, 9.5287) -> (4.5233, 9.5287) centre (4.5423, 9.5287) ccw
  arc A408 (4.5233, 9.365) -> (4.5614, 9.365) centre (4.5423, 9.365) ccw
  line L175 (4.0513, 9.8311) -> (4.5424, 9.8311)
  arc A409 (4.5424, 9.8121) -> (4.5424, 9.8502) centre (4.5424, 9.8311) ccw
  arc A410 (4.0513, 9.8502) -> (4.0513, 9.8121) centre (4.0513, 9.8311) ccw
  line L176 (4.5424, 9.8311) -> (4.5424, 10.0767)
  arc A411 (4.5614, 10.0767) -> (4.5233, 10.0767) centre (4.5423, 10.0767) ccw
  arc A412 (4.5233, 9.8311) -> (4.5614, 9.8311) centre (4.5423, 9.8311) ccw
  line L177 (4.5424, 10.0767) -> (4.4605, 10.0767)
  arc A413 (4.4605, 10.0957) -> (4.4605, 10.0576) centre (4.4605, 10.0767) ccw
  arc A414 (4.5424, 10.0576) -> (4.5424, 10.0957) centre (4.5424, 10.0767) ccw
  line L178 (4.0513, 10.6416) -> (4.0513, 10.437)
  arc A415 (4.0323, 10.437) -> (4.0704, 10.437) centre (4.0514, 10.437) ccw
  arc A416 (4.0704, 10.6416) -> (4.0323, 10.6416) centre (4.0514, 10.6416) ccw
  arc A417 (4.0513, 10.437) -> (4.1741, 10.3142) centre (4.1741, 10.437) ccw
  arc A418 (4.0704, 10.437) -> (4.0323, 10.437) centre (4.0514, 10.437) ccw
  arc A419 (4.1741, 10.2951) -> (4.1741, 10.3332) centre (4.1741, 10.3141) ccw
  line L179 (4.1741, 10.3142) -> (4.3787, 10.3142)
  arc A420 (4.3787, 10.2951) -> (4.3787, 10.3332) centre (4.3787, 10.3141) ccw
  arc A421 (4.1741, 10.3332) -> (4.1741, 10.2951) centre (4.1741, 10.3141) ccw
  arc A422 (4.3787, 10.3142) -> (4.3787, 10.6416) centre (4.3787, 10.4779) ccw
  arc A423 (4.3787, 10.3332) -> (4.3787, 10.2951) centre (4.3787, 10.3141) ccw
  arc A424 (4.3787, 10.6606) -> (4.3787, 10.6225) centre (4.3787, 10.6416) ccw
  line L180 (4.3787, 10.6416) -> (4.2968, 10.6416)
  arc A425 (4.2968, 10.6606) -> (4.2968, 10.6225) centre (4.2968, 10.6416) ccw
  arc A426 (4.3787, 10.6225) -> (4.3787, 10.6606) centre (4.3787, 10.6416) ccw
  line L181 (4.2968, 10.6416) -> (4.2968, 10.3142)
  arc A427 (4.2778, 10.3142) -> (4.3159, 10.3142) centre (4.2969, 10.3142) ccw
  arc A428 (4.3159, 10.6416) -> (4.2778, 10.6416) centre (4.2969, 10.6416) ccw
  line L182 (4.0513, 11.2755) -> (4.0513, 11.0709)
  arc A429 (4.0323, 11.0709) -> (4.0704, 11.0709) centre (4.0514, 11.0709) ccw
  arc A430 (4.0704, 11.2755) -> (4.0323, 11.2755) centre (4.0514, 11.2755) ccw
  arc A431 (4.0513, 11.0709) -> (4.1741, 10.9482) centre (4.1741, 11.071) ccw
  arc A432 (4.0704, 11.0709) -> (4.0323, 11.0709) centre (4.0514, 11.0709) ccw
  arc A433 (4.1741, 10.9291) -> (4.1741, 10.9672) centre (4.1741, 10.9482) ccw
  line L183 (4.1741, 10.9482) -> (4.3787, 10.9482)
  arc A434 (4.3787, 10.9291) -> (4.3787, 10.9672) centre (4.3787, 10.9482) ccw
  arc A435 (4.1741, 10.9672) -> (4.1741, 10.9291) centre (4.1741, 10.9482) ccw
  arc A436 (4.3787, 10.9482) -> (4.3787, 11.2755) centre (4.3787, 11.1119) ccw
  arc A437 (4.3787, 10.9672) -> (4.3787, 10.9291) centre (4.3787, 10.9482) ccw
  arc A438 (4.3787, 11.2946) -> (4.3787, 11.2565) centre (4.3787, 11.2756) ccw
  line L184 (4.3787, 11.2755) -> (4.2968, 11.2755)
  arc A439 (4.2968, 11.2946) -> (4.2968, 11.2565) centre (4.2968, 11.2756) ccw
  arc A440 (4.3787, 11.2565) -> (4.3787, 11.2946) centre (4.3787, 11.2756) ccw
  line L185 (4.2968, 11.2755) -> (4.2968, 10.9482)
  arc A441 (4.2778, 10.9482) -> (4.3159, 10.9482) centre (4.2969, 10.9482) ccw
  arc A442 (4.3159, 11.2755) -> (4.2778, 11.2755) centre (4.2969, 11.2755) ccw
  line L186 (4.0513, 11.6065) -> (4.5424, 11.6065)
  arc A443 (4.5424, 11.5875) -> (4.5424, 11.6256) centre (4.5424, 11.6066) ccw
  arc A444 (4.0513, 11.6256) -> (4.0513, 11.5875) centre (4.0513, 11.6066) ccw
  line L187 (4.5424, 11.6065) -> (4.5424, 11.8111)
  arc A445 (4.5614, 11.8111) -> (4.5233, 11.8111) centre (4.5423, 11.8111) ccw
  arc A446 (4.5233, 11.6065) -> (4.5614, 11.6065) centre (4.5423, 11.6065) ccw
  arc A447 (4.5424, 11.8111) -> (4.4196, 11.9339) centre (4.4196, 11.8111) ccw
  arc A448 (4.5233, 11.8111) -> (4.5614, 11.8111) centre (4.5423, 11.8111) ccw
  arc A449 (4.4196, 11.953) -> (4.4196, 11.9149) centre (4.4196, 11.9339) ccw
  line L188 (4.4196, 11.9339) -> (4.0513, 11.9339)
  arc A450 (4.0513, 11.953) -> (4.0513, 11.9149) centre (4.0513, 11.9339) ccw
  arc A451 (4.4196, 11.9149) -> (4.4196, 11.953) centre (4.4196, 11.9339) ccw
  line L189 (3.2413, 5.3721) -> (3.2413, 5.5767)
  arc A452 (3.2604, 5.5767) -> (3.2223, 5.5767) centre (3.2414, 5.5767) ccw
  arc A453 (3.2223, 5.3721) -> (3.2604, 5.3721) centre (3.2414, 5.3721) ccw
  arc A454 (3.2413, 5.5767) -> (2.8321, 5.5767) centre (3.0367, 5.5767) ccw
  arc A455 (3.2223, 5.5767) -> (3.2604, 5.5767) centre (3.2414, 5.5767) ccw
  arc A456 (2.813, 5.5767) -> (2.8511, 5.5767) centre (2.8321, 5.5767) ccw
  line L190 (2.8321, 5.5767) -> (2.8321, 5.3721)
  arc A457 (2.8131, 5.3721) -> (2.8512, 5.3721) centre (2.8321, 5.3721) ccw
  arc A458 (2.8512, 5.5767) -> (2.8131, 5.5767) centre (2.8321, 5.5767) ccw
  line L191 (2.8321, 5.3721) -> (3.5687, 5.3721)
  arc A459 (3.5687, 5.3531) -> (3.5687, 5.3912) centre (3.5687, 5.3722) ccw
  arc A460 (2.8321, 5.3912) -> (2.8321, 5.3531) centre (2.8321, 5.3722) ccw
  line L192 (3.5687, 5.3721) -> (3.5687, 5.5767)
  arc A461 (3.5878, 5.5767) -> (3.5497, 5.5767) centre (3.5688, 5.5767) ccw
  arc A462 (3.5497, 5.3721) -> (3.5878, 5.3721) centre (3.5688, 5.3721) ccw
  arc A463 (3.5687, 5.5767) -> (3.2413, 5.5767) centre (3.405, 5.5767) ccw
  arc A464 (3.5497, 5.5767) -> (3.5878, 5.5767) centre (3.5688, 5.5767) ccw
  arc A465 (3.2223, 5.5767) -> (3.2604, 5.5767) centre (3.2414, 5.5767) ccw
  line L193 (2.8321, 6.0886) -> (3.3232, 6.0886)
  arc A466 (3.3232, 6.0696) -> (3.3232, 6.1077) centre (3.3232, 6.0887) ccw
  arc A467 (2.8321, 6.1077) -> (2.8321, 6.0696) centre (2.8321, 6.0887) ccw
  line L194 (3.3232, 6.0886) -> (3.3232, 6.3342)
  arc A468 (3.3422, 6.3342) -> (3.3041, 6.3342) centre (3.3232, 6.3342) ccw
  arc A469 (3.3041, 6.0886) -> (3.3422, 6.0886) centre (3.3232, 6.0886) ccw
  line L195 (3.3232, 6.3342) -> (3.2413, 6.3342)
  arc A470 (3.2413, 6.3532) -> (3.2413, 6.3151) centre (3.2413, 6.3342) ccw
  arc A471 (3.3232, 6.3151) -> (3.3232, 6.3532) centre (3.3232, 6.3342) ccw
  line L196 (2.8321, 6.8991) -> (2.8321, 6.6944)
  arc A472 (2.8131, 6.6944) -> (2.8512, 6.6944) centre (2.8321, 6.6944) ccw
  arc A473 (2.8512, 6.8991) -> (2.8131, 6.8991) centre (2.8321, 6.8991) ccw
  arc A474 (2.8321, 6.6944) -> (2.9549, 6.5717) centre (2.9549, 6.6945) ccw
  arc A475 (2.8512, 6.6944) -> (2.8131, 6.6944) centre (2.8321, 6.6944) ccw
  arc A476 (2.9549, 6.5526) -> (2.9549, 6.5907) centre (2.9549, 6.5716) ccw
  line L197 (2.9549, 6.5717) -> (3.1595, 6.5717)
  arc A477 (3.1595, 6.5526) -> (3.1595, 6.5907) centre (3.1595, 6.5716) ccw
  arc A478 (2.9549, 6.5907) -> (2.9549, 6.5526) centre (2.9549, 6.5716) ccw
  arc A479 (3.1595, 6.5717) -> (3.1595, 6.8991) centre (3.1595, 6.7354) ccw
  arc A480 (3.1595, 6.5907) -> (3.1595, 6.5526) centre (3.1595, 6.5716) ccw
  arc A481 (3.1595, 6.9181) -> (3.1595, 6.88) centre (3.1595, 6.899) ccw
  line L198 (3.1595, 6.8991) -> (3.0776, 6.8991)
  arc A482 (3.0776, 6.9181) -> (3.0776, 6.88) centre (3.0776, 6.899) ccw
  arc A483 (3.1595, 6.88) -> (3.1595, 6.9181) centre (3.1595, 6.899) ccw
  line L199 (3.0776, 6.8991) -> (3.0776, 6.5717)
  arc A484 (3.0586, 6.5717) -> (3.0967, 6.5717) centre (3.0777, 6.5717) ccw
  arc A485 (3.0967, 6.8991) -> (3.0586, 6.8991) centre (3.0777, 6.8991) ccw
  line L200 (3.1186, 7.5289) -> (3.1186, 7.3448)
  arc A486 (3.0995, 7.3448) -> (3.1376, 7.3448) centre (3.1185, 7.3448) ccw
  arc A487 (3.1376, 7.5289) -> (3.0995, 7.5289) centre (3.1185, 7.5289) ccw
  arc A488 (2.8321, 7.3448) -> (3.1186, 7.3448) centre (2.9753, 7.3448) ccw
  arc A489 (2.8511, 7.3448) -> (2.813, 7.3448) centre (2.8321, 7.3448) ccw
  arc A490 (3.1376, 7.3448) -> (3.0995, 7.3448) centre (3.1185, 7.3448) ccw
  line L201 (2.8321, 7.3448) -> (2.8321, 7.5289)
  arc A491 (2.8512, 7.5289) -> (2.8131, 7.5289) centre (2.8321, 7.5289) ccw
  arc A492 (2.8131, 7.3448) -> (2.8512, 7.3448) centre (2.8321, 7.3448) ccw
  line L202 (2.8321, 7.5289) -> (3.2004, 7.5289)
  arc A493 (3.2004, 7.5099) -> (3.2004, 7.548) centre (3.2004, 7.529) ccw
  arc A494 (2.8321, 7.548) -> (2.8321, 7.5099) centre (2.8321, 7.529) ccw
  arc A495 (3.3232, 7.4062) -> (3.2004, 7.5289) centre (3.2004, 7.4061) ccw
  arc A496 (3.3041, 7.4062) -> (3.3422, 7.4062) centre (3.3232, 7.4062) ccw
  arc A497 (3.2004, 7.548) -> (3.2004, 7.5099) centre (3.2004, 7.529) ccw
  line L203 (3.3232, 7.4062) -> (3.3232, 7.2425)
  arc A498 (3.3041, 7.2425) -> (3.3422, 7.2425) centre (3.3232, 7.2425) ccw
  arc A499 (3.3422, 7.4062) -> (3.3041, 7.4062) centre (3.3232, 7.4062) ccw
  line L204 (2.8321, 7.8978) -> (3.5687, 7.8978)
  arc A500 (3.5687, 7.8788) -> (3.5687, 7.9169) centre (3.5687, 7.8979) ccw
  arc A501 (2.8321, 7.9169) -> (2.8321, 7.8788) centre (2.8321, 7.8979) ccw
  line L205 (3.3232, 8.2252) -> (3.0776, 7.8978)
  arc A502 (3.0624, 7.9093) -> (3.0929, 7.8864) centre (3.0777, 7.8979) ccw
  arc A503 (3.3384, 8.2138) -> (3.3079, 8.2366) centre (3.3232, 8.2252) ccw
  line L206 (2.8321, 8.2252) -> (3.1799, 8.0411)
  arc A504 (3.171, 8.0242) -> (3.1889, 8.0579) centre (3.18, 8.0411) ccw
  arc A505 (2.841, 8.242) -> (2.8232, 8.2084) centre (2.8321, 8.2252) ccw
  line L207 (2.9958, 8.498) -> (3.1595, 8.498)
  arc A506 (3.1595, 8.479) -> (3.1595, 8.5171) centre (3.1595, 8.498) ccw
  arc A507 (2.9958, 8.5171) -> (2.9958, 8.479) centre (2.9958, 8.498) ccw
  arc A508 (3.1595, 8.498) -> (3.1595, 8.8254) centre (3.1595, 8.6617) ccw
  arc A509 (3.1595, 8.5171) -> (3.1595, 8.479) centre (3.1595, 8.498) ccw
  arc A510 (3.1595, 8.8444) -> (3.1595, 8.8063) centre (3.1595, 8.8254) ccw
  line L208 (3.1595, 8.8254) -> (2.9958, 8.8254)
  arc A511 (2.9958, 8.8444) -> (2.9958, 8.8063) centre (2.9958, 8.8254) ccw
  arc A512 (3.1595, 8.8063) -> (3.1595, 8.8444) centre (3.1595, 8.8254) ccw
  arc A513 (2.9958, 8.8254) -> (2.9958, 8.498) centre (2.9958, 8.6617) ccw
  arc A514 (2.9958, 8.8063) -> (2.9958, 8.8444) centre (2.9958, 8.8254) ccw
  arc A515 (2.9958, 8.479) -> (2.9958, 8.5171) centre (2.9958, 8.498) ccw
  line L209 (3.3232, 9.1564) -> (2.9549, 9.1564)
  arc A516 (2.9549, 9.1754) -> (2.9549, 9.1373) centre (2.9549, 9.1563) ccw
  arc A517 (3.3232, 9.1373) -> (3.3232, 9.1754) centre (3.3232, 9.1563) ccw
  arc A518 (2.8321, 9.2791) -> (2.9549, 9.1564) centre (2.9549, 9.2792) ccw
  arc A519 (2.8512, 9.2791) -> (2.8131, 9.2791) centre (2.8321, 9.2791) ccw
  arc A520 (2.9549, 9.1373) -> (2.9549, 9.1754) centre (2.9549, 9.1563) ccw
  line L210 (2.8321, 9.2791) -> (2.8321, 9.4838)
  arc A521 (2.8512, 9.4838) -> (2.8131, 9.4838) centre (2.8321, 9.4838) ccw
  arc A522 (2.8131, 9.2791) -> (2.8512, 9.2791) centre (2.8321, 9.2791) ccw
  line L211 (2.8321, 9.4838) -> (3.3232, 9.4838)
  arc A523 (3.3232, 9.4647) -> (3.3232, 9.5028) centre (3.3232, 9.4838) ccw
  arc A524 (2.8321, 9.5028) -> (2.8321, 9.4647) centre (2.8321, 9.4838) ccw
  line L212 (3.3232, 9.7517) -> (3.3232, 9.9972)
  arc A525 (3.3422, 9.9972) -> (3.3041, 9.9972) centre (3.3232, 9.9972) ccw
  arc A526 (3.3041, 9.7517) -> (3.3422, 9.7517) centre (3.3232, 9.7517) ccw